Autodesk Fusion 360 part; units mm, degrees
(part 2 of 4)
sketch "v2" plane through (0, 0, 0) normal (0, 1, 0) x (1, 0, 0)
  line L0 (60.175, -2.525) -> (73.175, -2.525)
  line L1 (60.175, -16.525) -> (73.175, -16.525)
  line L2 (59.675, -3.025) -> (59.675, -16.025)
  line L3 (73.675, -3.025) -> (73.675, -16.025)
  arc A0 (60.175, -2.525) -> (59.675, -3.025) centre (60.175, -3.025) ccw
  arc A1 (73.675, -3.025) -> (73.175, -2.525) centre (73.175, -3.025) ccw
  arc A2 (59.675, -16.025) -> (60.175, -16.525) centre (60.175, -16.025) ccw
  arc A3 (73.175, -16.525) -> (73.675, -16.025) centre (73.175, -16.025) ccw
  line L4 (41.125, -10.145) -> (54.125, -10.145)
  line L5 (41.125, -24.145) -> (54.125, -24.145)
  line L6 (40.625, -10.645) -> (40.625, -23.645)
  line L7 (54.625, -10.645) -> (54.625, -23.645)
  arc A4 (41.125, -10.145) -> (40.625, -10.645) centre (41.125, -10.645) ccw
  arc A5 (54.625, -10.645) -> (54.125, -10.145) centre (54.125, -10.645) ccw
  arc A6 (40.625, -23.645) -> (41.125, -24.145) centre (41.125, -23.645) ccw
  arc A7 (54.125, -24.145) -> (54.625, -23.645) centre (54.125, -23.645) ccw
  line L8 (79.225, -13.955) -> (92.225, -13.955)
  line L9 (79.225, -27.955) -> (92.225, -27.955)
  line L10 (78.725, -14.455) -> (78.725, -27.455)
  line L11 (92.725, -14.455) -> (92.725, -27.455)
  arc A8 (79.225, -13.955) -> (78.725, -14.455) centre (79.225, -14.455) ccw
  arc A9 (92.725, -14.455) -> (92.225, -13.955) centre (92.225, -14.455) ccw
  arc A10 (78.725, -27.455) -> (79.225, -27.955) centre (79.225, -27.455) ccw
  arc A11 (92.225, -27.955) -> (92.725, -27.455) centre (92.225, -27.455) ccw
  line L12 (98.275, -15.86) -> (111.275, -15.86)
  line L13 (98.275, -29.86) -> (111.275, -29.86)
  line L14 (97.775, -16.36) -> (97.775, -29.36)
  line L15 (111.775, -16.36) -> (111.775, -29.36)
  arc A12 (98.275, -15.86) -> (97.775, -16.36) centre (98.275, -16.36) ccw
  arc A13 (111.775, -16.36) -> (111.275, -15.86) centre (111.275, -16.36) ccw
  arc A14 (97.775, -29.36) -> (98.275, -29.86) centre (98.275, -29.36) ccw
  arc A15 (111.275, -29.86) -> (111.775, -29.36) centre (111.275, -29.36) ccw
  line L16 (22.075, -19.67) -> (35.075, -19.67)
  line L17 (22.075, -33.67) -> (35.075, -33.67)
  line L18 (21.575, -20.17) -> (21.575, -33.17)
  line L19 (35.575, -20.17) -> (35.575, -33.17)
  arc A16 (22.075, -19.67) -> (21.575, -20.17) centre (22.075, -20.17) ccw
  arc A17 (35.575, -20.17) -> (35.075, -19.67) centre (35.075, -20.17) ccw
  arc A18 (21.575, -33.17) -> (22.075, -33.67) centre (22.075, -33.17) ccw
  arc A19 (35.075, -33.67) -> (35.575, -33.17) centre (35.075, -33.17) ccw
  line L20 (3.025, -21.575) -> (16.025, -21.575)
  line L21 (3.025, -35.575) -> (16.025, -35.575)
  line L22 (2.525, -22.075) -> (2.525, -35.075)
  line L23 (16.525, -22.075) -> (16.525, -35.075)
  arc A20 (3.025, -21.575) -> (2.525, -22.075) centre (3.025, -22.075) ccw
  arc A21 (16.525, -22.075) -> (16.025, -21.575) centre (16.025, -22.075) ccw
  arc A22 (2.525, -35.075) -> (3.025, -35.575) centre (3.025, -35.075) ccw
  arc A23 (16.025, -35.575) -> (16.525, -35.075) centre (16.025, -35.075) ccw
  line L24 (60.175, -21.575) -> (73.175, -21.575)
  line L25 (60.175, -35.575) -> (73.175, -35.575)
  line L26 (59.675, -22.075) -> (59.675, -35.075)
  line L27 (73.675, -22.075) -> (73.675, -35.075)
  arc A24 (60.175, -21.575) -> (59.675, -22.075) centre (60.175, -22.075) ccw
  arc A25 (73.675, -22.075) -> (73.175, -21.575) centre (73.175, -22.075) ccw
  arc A26 (59.675, -35.075) -> (60.175, -35.575) centre (60.175, -35.075) ccw
  arc A27 (73.175, -35.575) -> (73.675, -35.075) centre (73.175, -35.075) ccw
  line L28 (41.125, -29.195) -> (54.125, -29.195)
  line L29 (41.125, -43.195) -> (54.125, -43.195)
  line L30 (40.625, -29.695) -> (40.625, -42.695)
  line L31 (54.625, -29.695) -> (54.625, -42.695)
  arc A28 (41.125, -29.195) -> (40.625, -29.695) centre (41.125, -29.695) ccw
  arc A29 (54.625, -29.695) -> (54.125, -29.195) centre (54.125, -29.695) ccw
  arc A30 (40.625, -42.695) -> (41.125, -43.195) centre (41.125, -42.695) ccw
  arc A31 (54.125, -43.195) -> (54.625, -42.695) centre (54.125, -42.695) ccw
  line L32 (79.225, -33.005) -> (92.225, -33.005)
  line L33 (79.225, -47.005) -> (92.225, -47.005)
  line L34 (78.725, -33.505) -> (78.725, -46.505)
  line L35 (92.725, -33.505) -> (92.725, -46.505)
  arc A32 (79.225, -33.005) -> (78.725, -33.505) centre (79.225, -33.505) ccw
  arc A33 (92.725, -33.505) -> (92.225, -33.005) centre (92.225, -33.505) ccw
  arc A34 (78.725, -46.505) -> (79.225, -47.005) centre (79.225, -46.505) ccw
  arc A35 (92.225, -47.005) -> (92.725, -46.505) centre (92.225, -46.505) ccw
  line L36 (98.275, -34.91) -> (111.275, -34.91)
  line L37 (98.275, -48.91) -> (111.275, -48.91)
  line L38 (97.775, -35.41) -> (97.775, -48.41)
  line L39 (111.775, -35.41) -> (111.775, -48.41)
  arc A36 (98.275, -34.91) -> (97.775, -35.41) centre (98.275, -35.41) ccw
  arc A37 (111.775, -35.41) -> (111.275, -34.91) centre (111.275, -35.41) ccw
  arc A38 (97.775, -48.41) -> (98.275, -48.91) centre (98.275, -48.41) ccw
  arc A39 (111.275, -48.91) -> (111.775, -48.41) centre (111.275, -48.41) ccw
  line L40 (22.075, -38.72) -> (35.075, -38.72)
  line L41 (22.075, -52.72) -> (35.075, -52.72)
  line L42 (21.575, -39.22) -> (21.575, -52.22)
  line L43 (35.575, -39.22) -> (35.575, -52.22)
  arc A40 (22.075, -38.72) -> (21.575, -39.22) centre (22.075, -39.22) ccw
  arc A41 (35.575, -39.22) -> (35.075, -38.72) centre (35.075, -39.22) ccw
  arc A42 (21.575, -52.22) -> (22.075, -52.72) centre (22.075, -52.22) ccw
  arc A43 (35.075, -52.72) -> (35.575, -52.22) centre (35.075, -52.22) ccw
  line L44 (3.025, -40.625) -> (16.025, -40.625)
  line L45 (3.025, -54.625) -> (16.025, -54.625)
  line L46 (2.525, -41.125) -> (2.525, -54.125)
  line L47 (16.525, -41.125) -> (16.525, -54.125)
  arc A44 (3.025, -40.625) -> (2.525, -41.125) centre (3.025, -41.125) ccw
  arc A45 (16.525, -41.125) -> (16.025, -40.625) centre (16.025, -41.125) ccw
  arc A46 (2.525, -54.125) -> (3.025, -54.625) centre (3.025, -54.125) ccw
  arc A47 (16.025, -54.625) -> (16.525, -54.125) centre (16.025, -54.125) ccw
  line L48 (60.175, -40.625) -> (73.175, -40.625)
  line L49 (60.175, -54.625) -> (73.175, -54.625)
  line L50 (59.675, -41.125) -> (59.675, -54.125)
  line L51 (73.675, -41.125) -> (73.675, -54.125)
  arc A48 (60.175, -40.625) -> (59.675, -41.125) centre (60.175, -41.125) ccw
  arc A49 (73.675, -41.125) -> (73.175, -40.625) centre (73.175, -41.125) ccw
  arc A50 (59.675, -54.125) -> (60.175, -54.625) centre (60.175, -54.125) ccw
  arc A51 (73.175, -54.625) -> (73.675, -54.125) centre (73.175, -54.125) ccw
  line L52 (41.125, -48.245) -> (54.125, -48.245)
  line L53 (41.125, -62.245) -> (54.125, -62.245)
  line L54 (40.625, -48.745) -> (40.625, -61.745)
  line L55 (54.625, -48.745) -> (54.625, -61.745)
  arc A52 (41.125, -48.245) -> (40.625, -48.745) centre (41.125, -48.745) ccw
  arc A53 (54.625, -48.745) -> (54.125, -48.245) centre (54.125, -48.745) ccw
  arc A54 (40.625, -61.745) -> (41.125, -62.245) centre (41.125, -61.745) ccw
  arc A55 (54.125, -62.245) -> (54.625, -61.745) centre (54.125, -61.745) ccw
  line L56 (79.225, -52.055) -> (92.225, -52.055)
  line L57 (79.225, -66.055) -> (92.225, -66.055)
  line L58 (78.725, -52.555) -> (78.725, -65.555)
  line L59 (92.725, -52.555) -> (92.725, -65.555)
  arc A56 (79.225, -52.055) -> (78.725, -52.555) centre (79.225, -52.555) ccw
  arc A57 (92.725, -52.555) -> (92.225, -52.055) centre (92.225, -52.555) ccw
  arc A58 (78.725, -65.555) -> (79.225, -66.055) centre (79.225, -65.555) ccw
  arc A59 (92.225, -66.055) -> (92.725, -65.555) centre (92.225, -65.555) ccw
  line L60 (98.275, -53.96) -> (111.275, -53.96)
  line L61 (98.275, -67.96) -> (111.275, -67.96)
  line L62 (97.775, -54.46) -> (97.775, -67.46)
  line L63 (111.775, -54.46) -> (111.775, -67.46)
  arc A60 (98.275, -53.96) -> (97.775, -54.46) centre (98.275, -54.46) ccw
  arc A61 (111.775, -54.46) -> (111.275, -53.96) centre (111.275, -54.46) ccw
  arc A62 (97.775, -67.46) -> (98.275, -67.96) centre (98.275, -67.46) ccw
  arc A63 (111.275, -67.96) -> (111.775, -67.46) centre (111.275, -67.46) ccw
  line L64 (22.075, -57.77) -> (35.075, -57.77)
  line L65 (22.075, -71.77) -> (35.075, -71.77)
  line L66 (21.575, -58.27) -> (21.575, -71.27)
  line L67 (35.575, -58.27) -> (35.575, -71.27)
  arc A64 (22.075, -57.77) -> (21.575, -58.27) centre (22.075, -58.27) ccw
  arc A65 (35.575, -58.27) -> (35.075, -57.77) centre (35.075, -58.27) ccw
  arc A66 (21.575, -71.27) -> (22.075, -71.77) centre (22.075, -71.27) ccw
  arc A67 (35.075, -71.77) -> (35.575, -71.27) centre (35.075, -71.27) ccw
  line L68 (3.025, -59.675) -> (16.025, -59.675)
  line L69 (3.025, -73.675) -> (16.025, -73.675)
  line L70 (2.525, -60.175) -> (2.525, -73.175)
  line L71 (16.525, -60.175) -> (16.525, -73.175)
  arc A68 (3.025, -59.675) -> (2.525, -60.175) centre (3.025, -60.175) ccw
  arc A69 (16.525, -60.175) -> (16.025, -59.675) centre (16.025, -60.175) ccw
  arc A70 (2.525, -73.175) -> (3.025, -73.675) centre (3.025, -73.175) ccw
  arc A71 (16.025, -73.675) -> (16.525, -73.175) centre (16.025, -73.175) ccw
  line L72 (72.5575, -73.9625) -> (85.5575, -73.9625)
  line L73 (72.5575, -87.9625) -> (85.5575, -87.9625)
  line L74 (72.0575, -74.4625) -> (72.0575, -87.4625)
  line L75 (86.0575, -74.4625) -> (86.0575, -87.4625)
  arc A72 (72.5575, -73.9625) -> (72.0575, -74.4625) centre (72.5575, -74.4625) ccw
  arc A73 (86.0575, -74.4625) -> (85.5575, -73.9625) centre (85.5575, -74.4625) ccw
  arc A74 (72.0575, -87.4625) -> (72.5575, -87.9625) centre (72.5575, -87.4625) ccw
  arc A75 (85.5575, -87.9625) -> (86.0575, -87.4625) centre (85.5575, -87.4625) ccw
  line L76 (96.4107, -75.7169) -> (108.9677, -79.0815)
  line L77 (92.7872, -89.2398) -> (105.3442, -92.6045)
  line L78 (95.7983, -76.0704) -> (92.4336, -88.6274)
  line L79 (109.3213, -79.6939) -> (105.9566, -92.2509)
  arc A76 (96.4107, -75.7169) -> (95.7983, -76.0704) centre (96.2813, -76.1998) ccw
  arc A77 (109.3213, -79.6939) -> (108.9677, -79.0815) centre (108.8383, -79.5645) ccw
  arc A78 (92.4336, -88.6274) -> (92.7872, -89.2398) centre (92.9166, -88.7568) ccw
  arc A79 (105.3442, -92.6045) -> (105.9566, -92.2509) centre (105.4736, -92.1215) ccw
  line L80 (132.3373, -85.6651) -> (125.8373, -96.9234)
  line L81 (120.213, -78.6651) -> (113.713, -89.9234)
  line L82 (132.1543, -84.9821) -> (120.896, -78.4821)
  line L83 (125.1543, -97.1064) -> (113.896, -90.6064)
  arc A80 (132.3373, -85.6651) -> (132.1543, -84.9821) centre (131.9043, -85.4151) ccw
  arc A81 (125.1543, -97.1064) -> (125.8373, -96.9234) centre (125.4043, -96.6734) ccw
  arc A82 (120.896, -78.4821) -> (120.213, -78.6651) centre (120.646, -78.9151) ccw
  arc A83 (113.713, -89.9234) -> (113.896, -90.6064) centre (114.146, -90.1734) ccw
  line L84 (6.575, -19.575) -> (19.075, -19.575)
  line L85 (2.525, -41.125) -> (2.525, -54.125)
  line L86 (2.525, -60.175) -> (2.525, -73.175)
  line L87 (22.075, -71.77) -> (35.075, -71.77)
  line L88 (41.125, -62.245) -> (54.125, -62.245)
  line L89 (0.525, -41.125) -> (0.525, -54.125)
  line L90 (0.525, -60.175) -> (0.525, -74.675)
  line L91 (0.525, -22.075) -> (0.525, -35.075)
  line L92 (1.525, -75.675) -> (16.025, -75.675)
  line L93 (72.0575, -74.4625) -> (72.0575, -87.4625)
  line L94 (113.775, -54.46) -> (113.775, -65.0177)
  line L95 (113.775, -35.41) -> (113.775, -48.41)
  line L96 (113.775, -16.36) -> (113.775, -29.36)
  line L97 (25.625, -17.67) -> (38.125, -17.67)
  line L98 (44.675, -8.145) -> (57.175, -8.145)
  line L99 (60.175, -0.525) -> (73.175, -0.525)
  line L100 (76.175, -11.955) -> (88.675, -11.955)
  line L101 (95.225, -13.86) -> (107.725, -13.86)
  line L102 (132.1543, -84.9821) -> (120.896, -78.4821)
  line L103 (136.7533, -80.0163) -> (115.275, -67.6158)
  line L104 (137.1194, -81.3823) -> (127.5694, -97.9234)
  line L105 (68.5566, -88.749) -> (60.0623, -76.9247)
  line L106 (16.025, -75.675) -> (57.6258, -75.675)
  line L107 (124.5194, -103.2062) -> (127.5694, -97.9234)
  line L108 (113.775, -54.46) -> (113.775, -48.41)
  line L109 (113.775, -35.41) -> (113.775, -29.36)
  line L110 (0.525, -60.175) -> (0.525, -54.125)
  line L111 (0.525, -41.125) -> (0.525, -35.075)
  arc A84 (60.0623, -76.9247) -> (57.6258, -75.675) centre (57.6258, -78.675) ccw
  line L112 (6.575, -19.575) -> (3.025, -19.575)
  line L113 (0.525, -22.075) -> (0.525, -20.575)
  line L114 (1.525, -19.575) -> (3.025, -19.575)
  line L115 (19.575, -19.075) -> (19.575, -18.17)
  line L116 (20.075, -17.67) -> (25.625, -17.67)
  line L117 (38.625, -17.17) -> (38.625, -8.645)
  line L118 (39.125, -8.145) -> (44.675, -8.145)
  line L119 (57.675, -7.645) -> (57.675, -1.025)
  line L120 (58.175, -0.525) -> (60.175, -0.525)
  line L121 (75.675, -11.455) -> (75.675, -1.025)
  line L122 (75.175, -0.525) -> (73.175, -0.525)
  line L123 (88.675, -11.955) -> (94.225, -11.955)
  line L124 (94.725, -12.455) -> (94.725, -13.36)
  line L125 (107.725, -13.86) -> (112.775, -13.86)
  line L126 (113.775, -14.86) -> (113.775, -16.36)
  arc A85 (1.525, -19.575) -> (0.525, -20.575) centre (1.525, -20.575) ccw
  arc A86 (0.525, -74.675) -> (1.525, -75.675) centre (1.525, -74.675) ccw
  arc A87 (137.1194, -81.3823) -> (136.7533, -80.0163) centre (136.2533, -80.8823) ccw
  arc A88 (113.775, -14.86) -> (112.775, -13.86) centre (112.775, -14.86) ccw
  arc A89 (20.075, -17.67) -> (19.575, -18.17) centre (20.075, -18.17) ccw
  arc A90 (19.075, -19.575) -> (19.575, -19.075) centre (19.075, -19.075) ccw
  arc A91 (38.125, -17.67) -> (38.625, -17.17) centre (38.125, -17.17) ccw
  arc A92 (39.125, -8.145) -> (38.625, -8.645) centre (39.125, -8.645) ccw
  arc A93 (57.175, -8.145) -> (57.675, -7.645) centre (57.175, -7.645) ccw
  arc A94 (58.175, -0.525) -> (57.675, -1.025) centre (58.175, -1.025) ccw
  arc A95 (75.675, -1.025) -> (75.175, -0.525) centre (75.175, -1.025) ccw
  arc A96 (75.675, -11.455) -> (76.175, -11.955) centre (76.175, -11.455) ccw
  arc A97 (94.725, -12.455) -> (94.225, -11.955) centre (94.225, -12.455) ccw
  arc A98 (94.725, -13.36) -> (95.225, -13.86) centre (95.225, -13.36) ccw
  arc A99 (113.775, -65.0177) -> (115.275, -67.6158) centre (116.775, -65.0177) ccw
  line L127 (123.1533, -103.5722) -> (110.8977, -96.4964)
  arc A100 (123.1533, -103.5722) -> (124.5194, -103.2062) centre (123.6533, -102.7062) ccw
  line L128 (70.5283, -89.9625) -> (109.8625, -96.1307)
  arc A101 (68.5566, -88.749) -> (70.5283, -89.9625) centre (70.9931, -86.9987) ccw
  arc A102 (110.8977, -96.4964) -> (109.8625, -96.1307) centre (109.3977, -99.0945) ccw
  line L129 (16.025, -35.075) -> (22.075, -35.075) construction
  line L130 (22.075, -35.075) -> (22.075, -41.125) construction
  line L131 (22.075, -41.125) -> (16.025, -41.125) construction
  line L132 (16.025, -41.125) -> (16.025, -35.075) construction
  circle A103 centre (19.05, -38.1) radius 1
  line L133 (16.025, -54.125) -> (22.075, -54.125) construction
  line L134 (22.075, -54.125) -> (22.075, -60.175) construction
  line L135 (22.075, -60.175) -> (16.025, -60.175) construction
  line L136 (16.025, -60.175) -> (16.025, -54.125) construction
  circle A104 centre (19.05, -57.15) radius 1
  line L137 (92.225, -27.455) -> (98.275, -27.455) construction
  line L138 (98.275, -27.455) -> (98.275, -33.505) construction
  line L139 (98.275, -33.505) -> (92.225, -33.505) construction
  line L140 (92.225, -33.505) -> (92.225, -27.455) construction
  circle A105 centre (95.25, -30.48) radius 1
  line L141 (92.225, -46.505) -> (98.275, -46.505) construction
  line L142 (98.275, -46.505) -> (98.275, -52.555) construction
  line L143 (98.275, -52.555) -> (92.225, -52.555) construction
  line L144 (92.225, -52.555) -> (92.225, -46.505) construction
  circle A106 centre (95.25, -49.53) radius 1
  line L145 (66.675, -47.625) -> (66.675, -65.625) construction
  circle A107 centre (66.675, -65.625) radius 1
  line L146 (289.825, -35.575) -> (276.825, -35.575)
  arc A108 (238.225, -48.41) -> (238.725, -48.91) centre (238.725, -48.41) ccw
  arc A109 (251.725, -48.91) -> (252.225, -48.41) centre (251.725, -48.41) ccw
  arc A110 (238.725, -53.96) -> (238.225, -54.46) centre (238.725, -54.46) ccw
  arc A111 (238.725, -34.91) -> (238.225, -35.41) centre (238.725, -35.41) ccw
  line L147 (252.225, -35.41) -> (252.225, -48.41)
  line L148 (236.225, -35.41) -> (236.225, -48.41)
  line L149 (236.225, -35.41) -> (236.225, -29.36)
  arc A112 (252.225, -35.41) -> (251.725, -34.91) centre (251.725, -35.41) ccw
  line L150 (251.725, -29.86) -> (238.725, -29.86)
  line L151 (251.725, -27.455) -> (251.725, -33.505) construction
  line L152 (251.725, -34.91) -> (238.725, -34.91)
  line L153 (251.725, -46.505) -> (251.725, -52.555) construction
  line L154 (238.225, -35.41) -> (238.225, -48.41)
  arc A113 (238.225, -29.36) -> (238.725, -29.86) centre (238.725, -29.36) ccw
  line L155 (236.225, -54.46) -> (236.225, -48.41)
  arc A114 (252.225, -54.46) -> (251.725, -53.96) centre (251.725, -54.46) ccw
  line L156 (251.725, -48.91) -> (238.725, -48.91)
  line L157 (251.725, -53.96) -> (238.725, -53.96)
  arc A115 (251.725, -29.86) -> (252.225, -29.36) centre (251.725, -29.36) ccw
  line L158 (257.775, -33.505) -> (257.775, -27.455) construction
  line L159 (289.825, -2.525) -> (276.825, -2.525)
  line L160 (289.825, -16.525) -> (276.825, -16.525)
  line L161 (289.825, -21.575) -> (276.825, -21.575)
  arc A116 (276.325, -54.125) -> (276.825, -54.625) centre (276.825, -54.125) ccw
  arc A117 (257.275, -46.505) -> (257.775, -47.005) centre (257.775, -46.505) ccw
  arc A118 (257.775, -33.005) -> (257.275, -33.505) centre (257.775, -33.505) ccw
  line L162 (257.775, -52.555) -> (257.775, -46.505) construction
  arc A119 (257.775, -52.055) -> (257.275, -52.555) centre (257.775, -52.555) ccw
  line L163 (257.275, -33.505) -> (257.275, -46.505)
  arc A120 (276.825, -40.625) -> (276.325, -41.125) centre (276.825, -41.125) ccw
  arc A121 (270.775, -27.955) -> (271.275, -27.455) centre (270.775, -27.455) ccw
  line L164 (289.825, -40.625) -> (276.825, -40.625)
  line L165 (270.775, -52.055) -> (257.775, -52.055)
  line L166 (270.775, -47.005) -> (257.775, -47.005)
  line L167 (276.325, -41.125) -> (276.325, -54.125)
  line L168 (289.825, -0.525) -> (276.825, -0.525)
  arc A122 (276.325, -35.075) -> (276.825, -35.575) centre (276.825, -35.075) ccw
  arc A123 (279.4717, -89.9625) -> (281.4434, -88.749) centre (279.0069, -86.9987) ccw
  line L169 (270.775, -27.955) -> (257.775, -27.955)
  line L170 (290.325, -41.125) -> (290.325, -54.125)
  line L171 (289.825, -54.625) -> (276.825, -54.625)
  arc A124 (271.275, -52.555) -> (270.775, -52.055) centre (270.775, -52.555) ccw
  line L172 (271.275, -33.505) -> (271.275, -46.505)
  line L173 (270.775, -33.005) -> (257.775, -33.005)
  line L174 (257.275, -52.555) -> (257.275, -65.555)
  line L175 (236.225, -54.46) -> (236.225, -65.0177)
  arc A125 (271.275, -33.505) -> (270.775, -33.005) centre (270.775, -33.505) ccw
  line L176 (309.375, -29.695) -> (309.375, -42.695)
  line L177 (271.275, -52.555) -> (271.275, -65.555)
  line L178 (314.425, -39.22) -> (314.425, -52.22)
  line L179 (236.225, -16.36) -> (236.225, -29.36)
  line L180 (333.475, -41.125) -> (333.475, -54.125)
  line L181 (349.475, -41.125) -> (349.475, -54.125)
  line L182 (252.225, -54.46) -> (252.225, -67.46)
  arc A126 (270.775, -47.005) -> (271.275, -46.505) centre (270.775, -46.505) ccw
  arc A127 (257.275, -27.455) -> (257.775, -27.955) centre (257.775, -27.455) ccw
  line L183 (271.275, -14.455) -> (271.275, -27.455)
  line L184 (295.375, -29.695) -> (295.375, -42.695)
  line L185 (257.775, -27.455) -> (251.725, -27.455) construction
  line L186 (253.5893, -75.7169) -> (241.0323, -79.0815)
  line L187 (238.225, -54.46) -> (238.225, -67.46)
  line L188 (238.225, -16.36) -> (238.225, -29.36)
  line L189 (328.425, -39.22) -> (328.425, -52.22)
  line L190 (251.725, -67.96) -> (238.725, -67.96)
  line L191 (347.475, -41.125) -> (347.475, -54.125)
  circle A128 centre (254.75, -49.53) radius 1
  line L192 (257.275, -14.455) -> (257.275, -27.455)
  line L193 (279.4717, -89.9625) -> (240.1375, -96.1307)
  line L194 (251.725, -52.555) -> (257.775, -52.555) construction
  line L195 (251.725, -33.505) -> (257.775, -33.505) construction
  line L196 (257.2128, -89.2398) -> (244.6558, -92.6045)
  arc A129 (237.225, -13.86) -> (236.225, -14.86) centre (237.225, -14.86) ccw
  line L197 (252.225, -16.36) -> (252.225, -29.36)
  arc A130 (255.775, -11.955) -> (255.275, -12.455) centre (255.775, -12.455) ccw
  line L198 (333.975, -75.675) -> (292.3742, -75.675)
  arc A131 (241.0323, -79.0815) -> (240.6787, -79.6939) centre (241.1617, -79.5645) ccw
  line L199 (217.8457, -84.9821) -> (229.104, -78.4821)
  line L200 (229.787, -78.6651) -> (236.287, -89.9234)
  arc A132 (277.9425, -74.4625) -> (277.4425, -73.9625) centre (277.4425, -74.4625) ccw
  line L201 (212.8806, -81.3823) -> (222.4306, -97.9234)
  circle A133 centre (254.75, -30.48) radius 1
  line L202 (347.475, -41.125) -> (347.475, -54.125)
  arc A134 (295.375, -61.745) -> (295.875, -62.245) centre (295.875, -61.745) ccw
  arc A135 (229.787, -78.6651) -> (229.104, -78.4821) centre (229.354, -78.9151) ccw
  line L203 (261.325, -11.955) -> (255.775, -11.955)
  arc A136 (238.225, -67.46) -> (238.725, -67.96) centre (238.725, -67.46) ccw
  line L204 (276.325, -22.075) -> (276.325, -35.075)
  line L205 (257.775, -46.505) -> (251.725, -46.505) construction
  arc A137 (314.925, -57.77) -> (314.425, -58.27) centre (314.925, -58.27) ccw
  line L206 (213.2467, -80.0163) -> (234.725, -67.6158)
  line L207 (274.825, -0.525) -> (276.825, -0.525)
  line L208 (277.9425, -74.4625) -> (277.9425, -87.4625)
  arc A138 (295.375, -23.645) -> (295.875, -24.145) centre (295.875, -23.645) ccw
  line L209 (308.875, -62.245) -> (295.875, -62.245)
  arc A139 (274.825, -0.525) -> (274.325, -1.025) centre (274.825, -1.025) ccw
  arc A140 (276.325, -16.025) -> (276.825, -16.525) centre (276.825, -16.025) ccw
  arc A141 (263.9425, -87.4625) -> (264.4425, -87.9625) centre (264.4425, -87.4625) ccw
  arc A142 (308.875, -24.145) -> (309.375, -23.645) centre (308.875, -23.645) ccw
  circle A143 centre (283.325, -65.625) radius 1
  arc A144 (251.725, -67.96) -> (252.225, -67.46) centre (251.725, -67.46) ccw
  line L210 (240.6787, -79.6939) -> (244.0434, -92.2509)
  line L211 (236.225, -14.86) -> (236.225, -16.36)
  arc A145 (252.225, -16.36) -> (251.725, -15.86) centre (251.725, -16.36) ccw
  line L212 (254.775, -13.86) -> (242.275, -13.86)
  arc A146 (234.725, -67.6158) -> (236.225, -65.0177) centre (233.225, -65.0177) ccw
  line L213 (255.275, -12.455) -> (255.275, -13.36)
  arc A147 (257.775, -13.955) -> (257.275, -14.455) centre (257.775, -14.455) ccw
  arc A148 (290.325, -22.075) -> (289.825, -21.575) centre (289.825, -22.075) ccw
  line L214 (242.275, -13.86) -> (237.225, -13.86)
  arc A149 (276.825, -2.525) -> (276.325, -3.025) centre (276.825, -3.025) ccw
  line L215 (327.925, -57.77) -> (314.925, -57.77)
  arc A150 (254.775, -13.86) -> (255.275, -13.36) centre (254.775, -13.36) ccw
  line L216 (308.875, -62.245) -> (295.875, -62.245)
  line L217 (254.2017, -76.0704) -> (257.5664, -88.6274)
  arc A151 (238.725, -15.86) -> (238.225, -16.36) centre (238.725, -16.36) ccw
  arc A152 (213.2467, -80.0163) -> (212.8806, -81.3823) centre (213.7467, -80.8823) ccw
  arc A153 (289.825, -54.625) -> (290.325, -54.125) centre (289.825, -54.125) ccw
  arc A154 (257.275, -65.555) -> (257.775, -66.055) centre (257.775, -65.555) ccw
  line L218 (324.375, -17.67) -> (311.875, -17.67)
  arc A155 (308.875, -62.245) -> (309.375, -61.745) centre (308.875, -61.745) ccw
  line L219 (308.875, -24.145) -> (295.875, -24.145)
  line L220 (251.725, -15.86) -> (238.725, -15.86)
  arc A156 (276.825, -21.575) -> (276.325, -22.075) centre (276.825, -22.075) ccw
  line L221 (277.4425, -87.9625) -> (264.4425, -87.9625)
  line L222 (327.925, -71.77) -> (314.925, -71.77)
  line L223 (309.375, -10.645) -> (309.375, -23.645)
  line L224 (217.8457, -84.9821) -> (229.104, -78.4821)
  line L225 (327.925, -52.72) -> (314.925, -52.72)
  line L226 (327.925, -41.125) -> (333.975, -41.125) construction
  arc A157 (290.325, -41.125) -> (289.825, -40.625) centre (289.825, -41.125) ccw
  arc A158 (309.375, -48.745) -> (308.875, -48.245) centre (308.875, -48.745) ccw
  line L227 (329.925, -17.67) -> (324.375, -17.67)
  line L228 (217.6627, -85.6651) -> (224.1627, -96.9234)
  line L229 (327.925, -71.77) -> (314.925, -71.77)
  circle A159 centre (330.95, -38.1) radius 1
  arc A160 (333.475, -73.175) -> (333.975, -73.675) centre (333.975, -73.175) ccw
  arc A161 (327.925, -71.77) -> (328.425, -71.27) centre (327.925, -71.27) ccw
  line L230 (291.825, -0.525) -> (289.825, -0.525)
  arc A162 (289.825, -16.525) -> (290.325, -16.025) centre (289.825, -16.025) ccw
  line L231 (310.875, -8.145) -> (305.325, -8.145)
  arc A163 (295.875, -10.145) -> (295.375, -10.645) centre (295.875, -10.645) ccw
  arc A164 (348.475, -75.675) -> (349.475, -74.675) centre (348.475, -74.675) ccw
  arc A165 (346.975, -73.675) -> (347.475, -73.175) centre (346.975, -73.175) ccw
  arc A166 (292.325, -1.025) -> (291.825, -0.525) centre (291.825, -1.025) ccw
  line L232 (346.975, -73.675) -> (333.975, -73.675)
  arc A167 (311.375, -8.645) -> (310.875, -8.145) centre (310.875, -8.645) ccw
  line L233 (263.9425, -74.4625) -> (263.9425, -87.4625)
  arc A168 (257.2128, -89.2398) -> (257.5664, -88.6274) centre (257.0834, -88.7568) ccw
  line L234 (314.425, -58.27) -> (314.425, -71.27)
  line L235 (225.4806, -103.2062) -> (222.4306, -97.9234)
  arc A169 (295.875, -29.195) -> (295.375, -29.695) centre (295.875, -29.695) ccw
  line L236 (281.4434, -88.749) -> (289.9377, -76.9247)
  line L237 (327.925, -19.67) -> (314.925, -19.67)
  line L238 (277.9425, -74.4625) -> (277.9425, -87.4625)
  arc A170 (236.104, -90.6064) -> (236.287, -89.9234) centre (235.854, -90.1734) ccw
  arc A171 (309.375, -29.695) -> (308.875, -29.195) centre (308.875, -29.695) ccw
  arc A172 (264.4425, -73.9625) -> (263.9425, -74.4625) centre (264.4425, -74.4625) ccw
  line L239 (226.8467, -103.5722) -> (239.1023, -96.4964)
  arc A173 (292.3742, -75.675) -> (289.9377, -76.9247) centre (292.3742, -78.675) ccw
  line L240 (276.325, -3.025) -> (276.325, -16.025)
  line L241 (224.8457, -97.1064) -> (236.104, -90.6064)
  line L242 (333.975, -35.075) -> (327.925, -35.075) construction
  arc A174 (289.825, -35.575) -> (290.325, -35.075) centre (289.825, -35.075) ccw
  line L243 (277.4425, -73.9625) -> (264.4425, -73.9625)
  arc A175 (225.4806, -103.2062) -> (226.8467, -103.5722) centre (226.3467, -102.7062) ccw
  line L244 (327.925, -38.72) -> (314.925, -38.72)
  arc A176 (254.2017, -76.0704) -> (253.5893, -75.7169) centre (253.7187, -76.1998) ccw
  arc A177 (314.925, -19.67) -> (314.425, -20.17) centre (314.925, -20.17) ccw
  line L245 (295.375, -10.645) -> (295.375, -23.645)
  arc A178 (314.425, -52.22) -> (314.925, -52.72) centre (314.925, -52.22) ccw
  arc A179 (240.1375, -96.1307) -> (239.1023, -96.4964) centre (240.6023, -99.0945) ccw
  arc A180 (217.8457, -84.9821) -> (217.6627, -85.6651) centre (218.0957, -85.4151) ccw
  line L246 (290.325, -22.075) -> (290.325, -35.075)
  arc A181 (270.775, -66.055) -> (271.275, -65.555) centre (270.775, -65.555) ccw
  line L247 (295.375, -48.745) -> (295.375, -61.745)
  line L248 (308.875, -29.195) -> (295.875, -29.195)
  arc A182 (308.875, -43.195) -> (309.375, -42.695) centre (308.875, -42.695) ccw
  arc A183 (314.425, -71.27) -> (314.925, -71.77) centre (314.925, -71.27) ccw
  line L249 (273.825, -11.955) -> (261.325, -11.955)
  line L250 (349.475, -22.075) -> (349.475, -20.575)
  arc A184 (327.925, -33.67) -> (328.425, -33.17) centre (327.925, -33.17) ccw
  line L251 (270.775, -66.055) -> (257.775, -66.055)
  arc A185 (295.875, -48.245) -> (295.375, -48.745) centre (295.875, -48.745) ccw
  line L252 (283.325, -47.625) -> (283.325, -65.625) construction
  line L253 (328.425, -58.27) -> (328.425, -71.27)
  arc A186 (271.275, -14.455) -> (270.775, -13.955) centre (270.775, -14.455) ccw
  arc A187 (273.825, -11.955) -> (274.325, -11.455) centre (273.825, -11.455) ccw
  arc A188 (347.475, -22.075) -> (346.975, -21.575) centre (346.975, -22.075) ccw
  arc A189 (277.4425, -87.9625) -> (277.9425, -87.4625) centre (277.4425, -87.4625) ccw
  arc A190 (314.425, -33.17) -> (314.925, -33.67) centre (314.925, -33.17) ccw
  line L254 (308.875, -48.245) -> (295.875, -48.245)
  arc A191 (328.425, -20.17) -> (327.925, -19.67) centre (327.925, -20.17) ccw
  line L255 (346.975, -59.675) -> (333.975, -59.675)
  line L256 (274.325, -11.455) -> (274.325, -1.025)
  line L257 (328.425, -20.17) -> (328.425, -33.17)
  arc A192 (295.375, -42.695) -> (295.875, -43.195) centre (295.875, -42.695) ccw
  line L258 (333.475, -60.175) -> (333.475, -73.175)
  line L259 (270.775, -13.955) -> (257.775, -13.955)
  line L260 (308.875, -43.195) -> (295.875, -43.195)
  line L261 (327.925, -35.075) -> (327.925, -41.125) construction
  line L262 (327.925, -60.175) -> (333.975, -60.175) construction
  line L263 (309.375, -48.745) -> (309.375, -61.745)
  arc A193 (333.975, -21.575) -> (333.475, -22.075) centre (333.975, -22.075) ccw
  arc A194 (224.1627, -96.9234) -> (224.8457, -97.1064) centre (224.5957, -96.6734) ccw
  arc A195 (314.925, -38.72) -> (314.425, -39.22) centre (314.925, -39.22) ccw
  arc A196 (244.0434, -92.2509) -> (244.6558, -92.6045) centre (244.5264, -92.1215) ccw
  arc A197 (347.475, -60.175) -> (346.975, -59.675) centre (346.975, -60.175) ccw
  arc A198 (333.475, -54.125) -> (333.975, -54.625) centre (333.975, -54.125) ccw
  line L264 (346.975, -35.575) -> (333.975, -35.575)
  line L265 (346.975, -40.625) -> (333.975, -40.625)
  arc A199 (292.325, -7.645) -> (292.825, -8.145) centre (292.825, -7.645) ccw
  line L266 (347.475, -60.175) -> (347.475, -73.175)
  arc A200 (330.425, -19.075) -> (330.925, -19.575) centre (330.925, -19.075) ccw
  circle A201 centre (330.95, -57.15) radius 1
  arc A202 (290.325, -3.025) -> (289.825, -2.525) centre (289.825, -3.025) ccw
  line L267 (305.325, -8.145) -> (292.825, -8.145)
  line L268 (347.475, -60.175) -> (347.475, -73.175)
  line L269 (290.325, -3.025) -> (290.325, -16.025)
  arc A203 (328.425, -39.22) -> (327.925, -38.72) centre (327.925, -39.22) ccw
  line L270 (314.425, -20.17) -> (314.425, -33.17)
  line L271 (292.325, -7.645) -> (292.325, -1.025)
  line L272 (333.475, -22.075) -> (333.475, -35.075)
  arc A204 (333.975, -59.675) -> (333.475, -60.175) centre (333.975, -60.175) ccw
  line L273 (349.475, -41.125) -> (349.475, -35.075)
  arc A205 (347.475, -41.125) -> (346.975, -40.625) centre (346.975, -41.125) ccw
  line L274 (349.475, -22.075) -> (349.475, -35.075)
  line L275 (346.975, -21.575) -> (333.975, -21.575)
  line L276 (327.925, -33.67) -> (314.925, -33.67)
  line L277 (311.375, -17.17) -> (311.375, -8.645)
  arc A206 (328.425, -58.27) -> (327.925, -57.77) centre (327.925, -58.27) ccw
  line L278 (349.475, -60.175) -> (349.475, -54.125)
  line L279 (327.925, -54.125) -> (327.925, -60.175) construction
  line L280 (349.475, -60.175) -> (349.475, -74.675)
  arc A207 (346.975, -35.575) -> (347.475, -35.075) centre (346.975, -35.075) ccw
  arc A208 (327.925, -52.72) -> (328.425, -52.22) centre (327.925, -52.22) ccw
  arc A209 (330.425, -18.17) -> (329.925, -17.67) centre (329.925, -18.17) ccw
  arc A210 (309.375, -10.645) -> (308.875, -10.145) centre (308.875, -10.645) ccw
  arc A211 (346.975, -54.625) -> (347.475, -54.125) centre (346.975, -54.125) ccw
  arc A212 (333.975, -40.625) -> (333.475, -41.125) centre (333.975, -41.125) ccw
  arc A213 (333.475, -35.075) -> (333.975, -35.575) centre (333.975, -35.075) ccw
  line L281 (333.975, -41.125) -> (333.975, -35.075) construction
  line L282 (346.975, -54.625) -> (333.975, -54.625)
  line L283 (348.475, -75.675) -> (333.975, -75.675)
  line L284 (343.425, -19.575) -> (330.925, -19.575)
  line L285 (333.975, -60.175) -> (333.975, -54.125) construction
  line L286 (348.475, -19.575) -> (346.975, -19.575)
  line L287 (308.875, -10.145) -> (295.875, -10.145)
  arc A214 (311.375, -17.17) -> (311.875, -17.67) centre (311.875, -17.17) ccw
  line L288 (347.475, -22.075) -> (347.475, -35.075)
  arc A215 (349.475, -20.575) -> (348.475, -19.575) centre (348.475, -20.575) ccw
  line L289 (343.425, -19.575) -> (346.975, -19.575)
  line L290 (330.425, -19.075) -> (330.425, -18.17)
  line L291 (333.975, -54.125) -> (327.925, -54.125) construction
  point P0 (19.575, -19.575)
  point P1 (57.675, -8.145)
  point P2 (94.725, -13.86)
  point P3 (75.675, -11.955)
  point P4 (38.625, -17.67)
  point P5 (311.375, -17.67)
  point P6 (274.325, -11.955)
  point P7 (292.325, -8.145)
  point P8 (255.275, -13.86)
  point P9 (330.425, -19.575)
  dimension "d52" = 4
  dimension "d55" = 3
  dimension "d56" = 2
  dimension "d57" = 2
  dimension "d58" = 2
  dimension "d59" = 2
  dimension "d60" = 2
  dimension "d61" = 1
  dimension "d62" = 1
  dimension "d64" = 1
  dimension "d65" = 1
  dimension "d66" = 0.5
  dimension "d68" = 0.5
  dimension "d69" = 0.5
  dimension "d70" = 0.5
  dimension "d71" = 0.5
  dimension "d72" = 0.5
  dimension "d73" = 0.5
  dimension "d74" = 0.5
  dimension "d75" = 0.5
  dimension "d76" = 0.5
  dimension "d78" = 3
  dimension "d79" = 2
  dimension "d82" = 6.6
  dimension "d83" = 2
  dimension "d84" = 2
  dimension "d85" = 2
  dimension "d112" = 2
  dimension "d114" = 6.6
  dimension "d115" = 1
  dimension "d120" = 3
  dimension "d121" = 3
  dimension "d122" = 2
  dimension "d123" = 2
  dimension "d124" = 2
  dimension "d125" = 2
  dimension "d126" = 2
  dimension "d127" = 18
  dimension "d128" = 2
  constraint parallel L92 L106
  constraint parallel L104 L107
  constraint parallel L95 L108
  constraint parallel L96 L109
  constraint perpendicular L92 L110
  constraint parallel L91 L111
  constraint tangent L105 A84
  constraint tangent L106 A84
  constraint perpendicular L22 L112
  constraint perpendicular L112 L113
  constraint perpendicular L91 L114
  constraint perpendicular L97 L115
  constraint perpendicular L115 L116
  constraint perpendicular L98 L117
  constraint perpendicular L117 L118
  constraint perpendicular L99 L119
  constraint perpendicular L7 L120
  constraint perpendicular L0 L121
  constraint perpendicular L121 L122
  constraint perpendicular L121 L123
  constraint perpendicular L123 L124
  constraint perpendicular L96 L125
  constraint perpendicular L101 L126
  constraint tangent L113 A85
  constraint tangent L114 A85
  constraint tangent L90 A86
  constraint tangent L92 A86
  constraint tangent L103 A87
  constraint tangent L104 A87
  constraint tangent L125 A88
  constraint tangent L126 A88
  constraint tangent L115 A89
  constraint tangent L116 A89
  constraint coincident P0 L84
  constraint coincident P0 L115
  constraint tangent L84 A90
  constraint tangent L115 A90
  constraint coincident P4 L97
  constraint coincident P4 L117
  constraint tangent L97 A91
  constraint tangent L117 A91
  constraint tangent L117 A92
  constraint tangent L118 A92
  constraint coincident P1 L98
  constraint coincident P1 L119
  constraint tangent L98 A93
  constraint tangent L119 A93
  constraint tangent L119 A94
  constraint tangent L120 A94
  constraint tangent L121 A95
  constraint tangent L122 A95
  constraint coincident P3 L100
  constraint coincident P3 L121
  constraint tangent L100 A96
  constraint tangent L121 A96
  constraint tangent L123 A97
  constraint tangent L124 A97
  constraint coincident P2 L101
  constraint coincident P2 L124
  constraint tangent L101 A98
  constraint tangent L124 A98
  constraint tangent L94 A99
  constraint tangent L103 A99
  constraint parallel L97 L106
  constraint tangent L127 A100
  constraint tangent L107 A100
  constraint tangent L105 A101
  constraint tangent L128 A101
  constraint tangent L128 A102
  constraint tangent L127 A102
  constraint horizontal L129
  constraint vertical L130
  constraint horizontal L131
  constraint vertical L132
  constraint coincident A23.centre L129.start
  constraint horizontal L133
  constraint vertical L134
  constraint horizontal L135
  constraint vertical L136
  constraint horizontal L137
  constraint vertical L138
  constraint horizontal L139
  constraint vertical L140
  constraint horizontal L141
  constraint vertical L142
  constraint horizontal L143
  constraint vertical L144
  constraint perpendicular L49 L145
  constraint coincident L145.end A107.centre
  measures "d52" distance of A74.centre L105
  measures "d55" radius of A84
  measures "d56" distance of L18 P0
  measures "d57" distance of L6 P4
  measures "d58" distance of L2 P1
  measures "d59" distance of L3 P3
  measures "d60" distance of L11 P2
  measures "d61" radius of A85
  measures "d62" radius of A86
  measures "d64" radius of A87
  measures "d65" radius of A88
  measures "d66" radius of A89
  measures "d68" radius of A90
  measures "d69" radius of A91
  measures "d70" radius of A92
  measures "d71" radius of A93
  measures "d72" radius of A94
  measures "d73" radius of A95
  measures "d74" radius of A96
  measures "d75" radius of A97
  measures "d76" radius of A98
  measures "d78" radius of A99
  measures "d79" distance of L69 L92
  measures "d82" distance of L82 L103
  measures "d83" distance of L16 L97
  measures "d84" distance of L4 L98
  measures "d85" distance of L0 L99
  measures "d112" distance of L80 L104
  measures "d114" distance of L83 L127
  measures "d115" radius of A100
  measures "d120" radius of A101
  measures "d121" radius of A102
  measures "d122" vertical distance of L73.start L128.start
  measures "d123" diameter of A103
  measures "d124" diameter of A104
  measures "d125" diameter of A105
  measures "d126" diameter of A106
  measures "d127" distance of L145.start L145.end
  measures "d128" diameter of A107
extrude "Extrude2" add sketch "v2" along normal blind 1 separate body makes body 3 at (44.7753, 0, 69.73) makes body 4 at (305.2247, 0, 69.73)
move_body "Move2" bodies 3 4 to x (1, 0, 0) y (0, 1, 0) z (0, 0, 1) at (0, 0, 170)